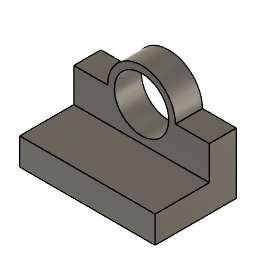
ex 3 (Autodesk Fusion 360 design; units mm, degrees)
part number: 2026-04-16-18-15-43-960
Autodesk Fusion 360 part; units mm, degrees
sketch "Sketch1" plane through (0, 0, 0) normal (0, 1, 0) x (1, 0, 0)
  line L0 (-50, -10) -> (50, -10)
  line L1 (50, -10) -> (50, -55)
  line L2 (50, -55) -> (-50, -55)
  line L3 (-50, -55) -> (-50, -10)
  circle A0 centre (0, -55) radius 20
  circle A1 centre (0, -55) radius 25
  dimension "d1" = 100
  dimension "d2" = 45
  dimension "d4" = 50
  constraint horizontal L0
  constraint perpendicular L0 L1
  constraint perpendicular L1 L2
  constraint perpendicular L0 L3
  constraint midpoint L2 A0.centre
  constraint concentric A0 A1
  measures "d1" distance of L0.start L0.end
  measures "d2" distance of L0.end L1.end
  measures "d4" diameter of A1
extrude "Extrude1" add sketch "Sketch1" along normal blind 20 contours L0 L1 L2 L3 A1 | L2 A0 A1 | L2 A0 A1
sketch "Sketch2" plane through (0, 0, 10) normal (0, 0, -1) x (1, 0, 0)
  line L0 (50, 0) -> (-50, 0)
  line L1 (-50, 0) -> (-50, -20)
  line L2 (-50, -20) -> (50, -20)
  line L3 (50, -20) -> (50, 0)
  line L4 (-50, 0) -> (-50, 40)
  line L5 (-50, 40) -> (50, 40)
  line L6 (50, 40) -> (50, 0)
  dimension "d7" = 40
  constraint coincident L0.end L1.start
  constraint perpendicular L0 L4
  constraint perpendicular L4 L5
  constraint coincident L0.start L3.end
  constraint perpendicular L0 L6
  measures "d7" distance of L0.end L4.end
extrude "Extrude2" add sketch "Sketch2" against normal blind 20 contours L0 L4 L5 L6
